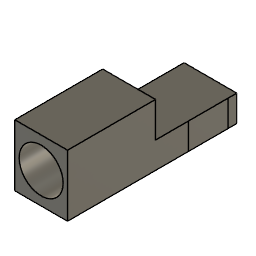
BoTech.StarClock.PowerSupply.Led (Autodesk Fusion 360 design; units mm, degrees)
Autodesk Fusion 360 part; units mm, degrees
note: some values were not read from the file. Set by a fixed rule: which sketch regions a step uses.
sketch "Skizze1" plane through (0, 0, 0) normal (0, 0, 1) x (1, 0, 0)
  circle A0 centre (0, 0) radius 3
  line L0 (2.5981, 1.5) -> (-2.5981, 1.5)
  circle A1 centre (0, 0) radius 2
  line L1 (-2.5981, 1.5) -> (-2.5981, 1)
  line L2 (-2.5981, 1) -> (-2.8284, 1)
  line L3 (-2.5981, 1) -> (2.8284, 1)
  line L4 (3, 0) -> (4.5, 0)
  line L5 (4.5, 0) -> (4.5, 1)
  line L6 (4.5, 1) -> (2.8284, 1)
  line L7 (-3, 0) -> (-4.5, 0)
  line L8 (-4.5, 0) -> (-4.5, 1)
  line L9 (-4.5, 1) -> (-2.8284, 1)
  line L10 (0, -3) -> (0, -4.5)
  line L11 (0, -4.5) -> (4.5, -4.5)
  line L12 (4.5, -4.5) -> (4.5, 0)
  line L13 (-4.5, 0) -> (-4.5, -4.5)
  line L14 (-4.5, -4.5) -> (0, -4.5)
  circle A2 centre (0, 0) radius 1.75
  line L15 (0, 1.75) -> (0, -8.25)
  line L16 (0, -8.25) -> (0, -18.25)
  line L17 (0, -8.25) -> (-4.5, -8.25)
  line L18 (-4.5, -8.25) -> (-4.5, -4.5)
  line L19 (0, -8.25) -> (4.5, -8.25)
  line L20 (4.5, -8.25) -> (4.5, -4.5)
  line L21 (4.5, -8.25) -> (4.4512, -8.25)
  line L22 (4.5, -8.25) -> (-4.5, -8.25)
  line L23 (-4.5, -8.25) -> (-4.5, -18.25)
  line L24 (-4.5, -18.25) -> (4.5, -18.25)
  line L25 (4.5, -18.25) -> (4.5, -8.25)
  line L26 (0, 0) -> (1.5, 0)
  line L27 (1.5, 0) -> (1.5, 1)
  line L28 (1.5, 0) -> (1.5, -18.25)
  line L29 (0, 0) -> (-1.5, 0)
  line L30 (-1.5, 0) -> (-1.5, 1)
  line L31 (-1.5, 0) -> (-1.5, -18.25)
  dimension "d2" = 6
  dimension "d3" = 0.5
  dimension "d4" = 1.5
  dimension "d5" = 1.5
  dimension "d6" = 1.5
  dimension "d7" = 4
  dimension "d8" = 3.5
  dimension "d19" = 10
  dimension "d20" = 10
  dimension "d21" = 9
  dimension "d22" = 10
  dimension "d32" = 1.5
  dimension "d33" = 1.5
  constraint concentric A0 A1
  constraint coincident L0.start A0
  constraint horizontal L0
  constraint coincident L0.end A0
  constraint perpendicular L0 L1
  constraint coincident A0 L2.end
  constraint perpendicular L1 L2
  constraint coincident A0 L3.end
  constraint perpendicular L1 L3
  constraint coincident A0 L4.start
  constraint parallel L3 L4
  constraint perpendicular L4 L5
  constraint perpendicular L5 L6
  constraint coincident A0 L7.start
  constraint parallel L2 L7
  constraint perpendicular L7 L8
  constraint perpendicular L8 L9
  constraint coincident A0 L10.start
  constraint perpendicular L7 L10
  constraint perpendicular L10 L11
  constraint perpendicular L7 L13
  constraint perpendicular L10 L14
  constraint concentric A0 A2
  constraint coincident A2 L15.start
  constraint perpendicular L14 L15
  constraint perpendicular L14 L16
  constraint perpendicular L15 L17
  constraint perpendicular L17 L18
  constraint perpendicular L15 L19
  constraint perpendicular L11 L20
  constraint coincident L19 L21.end
  constraint perpendicular L20 L21
  constraint horizontal L22
  constraint vertical L23
  constraint horizontal L24
  constraint vertical L25
  constraint coincident A0.centre A1.centre
  constraint parallel L3 L26
  constraint coincident L3 L27.end
  constraint perpendicular L3 L27
  constraint coincident L24 L28.end
  constraint perpendicular L24 L28
  constraint perpendicular L15 L29
  constraint coincident L3 L30.end
  constraint perpendicular L3 L30
  constraint coincident L24 L31.end
  constraint perpendicular L24 L31
  measures "d2" diameter of A0
  measures "d3" distance of L0.end L1.end
  measures "d4" distance of L4.start L4.end
  measures "d5" distance of L7.start L7.end
  measures "d6" distance of L10.start L10.end
  measures "d7" diameter of A1
  measures "d8" diameter of A2
  measures "d19" distance of L15.start L15.end
  measures "d20" distance of L15.end L16.end
  measures "d21" distance of L19.end L17.end
  measures "d22" distance of L19.end L24.end
  measures "d32" distance of A0.centre L26.end
  measures "d33" distance of A0.centre L29.end
extrude "Extrusion2" add sketch "Skizze1" along normal blind 2 contours L0 A1 L3 A2 | A1 L3 A2 L27 L28 | A1 A2 L15 L28 | L0 A1 A2 | L3 A2 L27 | A1 A2 L15 L31 | A2 L27 L28 | A2 L15 L26 L28 | L0 A1 L3 A2 | L0 L3 A2 L15 | L0 A2 L15 | L3 A2 L15 L26 L27 | A1 L3 A2 L30 L31 | A2 L15 L29 L31 | L0 A2 L15 | L0 L3 A2 L15 | L3 A2 L15 L29 L30 | A2 L30 L31 | L3 A2 L30
extrude "Extrusion5" add sketch "Skizze1" along normal blind 3 from surface at 2 contours A0 A1 L3 L28 | A0 L4 L11 L12 L28 | A0 L4 L5 L6 | A0 L10 L11 L15 L28 | A0 A1 L15 L28 | A1 L3 A2 L27 L28 | A0 L10 L14 L15 L31 | A0 A1 L15 L31 | A1 A2 L15 L28 | L11 L15 L19 L22 L28 | L11 L19 L20 L21 L22 L28 | L3 A2 L27 | L14 L15 L17 L22 L31 | A1 A2 L15 L31 | A2 L27 L28 | A2 L15 L26 L28 | L3 A2 L15 L26 L27 | A2 L15 L29 L31 | L3 A2 L15 L29 L30 | L3 A2 L30
extrude "Extrusion6" add sketch "Skizze1" along normal blind 7 from surface at 2 contours L16 L19 L22 L24 L28 | L19 L21 L22 L24 L25 L28 | L16 L17 L22 L24 L31
sketch "Skizze2" plane through (0, -18.25, 0) normal (0, -1, 0) x (1, 0, 0)
  line L0 (-1.5, 2) -> (4.5, 2)
  line L1 (4.5, 9) -> (-1.5, 9)
  circle A0 centre (1.5, 5.5) radius 2.5
  line L2 (4.5, 2) -> (4.5, 9)
  line L3 (-1.5, 9) -> (-1.5, 2)
  dimension "d29" = 5
  measures "d29" diameter of A0
extrude "Extrusion7" cut sketch "Skizze2" against normal blind 9.5 contours A0
